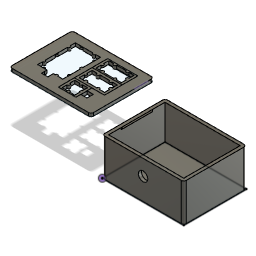
feather_case (Autodesk Fusion 360 design; units mm, degrees)
Autodesk Fusion 360 part; units mm, degrees
sketch "Base" plane through (0, 0, 0) normal (0, 1, 0) x (1, 0, 0) in component "Top"
  line L0 (0, 0) -> (130, 0)
  line L1 (130, 0) -> (130, 100)
  line L2 (130, 100) -> (0, 100)
  line L3 (0, 100) -> (0, 0)
  dimension "d6" = 130
  dimension "d7" = 100
  constraint horizontal L0
  constraint vertical L1
  constraint horizontal L2
  constraint vertical L3
  constraint coincident L0.start L3.end
  measures "d6" distance of L0.start L0.end
  measures "d7" distance of L0.start L2.end
extrude "Extrude1" add sketch "Base" along normal blind 60 makes body 1 in component "Top"
fillet "Fillet1" radius 4 4 edges at (130, 30, 0) (0, 30, 0) (130, 30, -100) (0, 30, -100) on bodies 1 in component "Top"
shell "Shell1" thickness 5 removed faces 1 at (85.3333, 60, -33.3333) on bodies 1 in component "Top"
sketch "Knob" plane through (5, 0, 0) normal (1, 0, 0) x (0, 0, -1) in component "Top"
  line L0 (95, 60) -> (5, 60)
  line L1 (5, 5) -> (95, 5)
  line L2 (25, 60) -> (75, 60)
  line L3 (75, 60) -> (75, 57)
  line L4 (75, 57) -> (25, 57)
  line L5 (25, 57) -> (25, 60)
  line L6 (50, 60) -> (50, 57) construction
  line L7 (5, 60) -> (5, 5)
  line L8 (95, 5) -> (95, 60)
  dimension "d12" = 50
  dimension "d13" = 3
  constraint horizontal L2
  constraint vertical L3
  constraint horizontal L4
  constraint vertical L5
  constraint coincident L0 L2.start
  constraint midpoint L0 L6.start
  constraint midpoint L4 L6.end
  constraint vertical L6
  measures "d12" distance of L3.end L4.end
  measures "d13" distance of L2.end L3.end
extrude "Extrude2" add sketch "Knob" along normal blind 6 draft -45 contours L0 L2 L3 L4 L5 bodies 1 in component "Top"
ref_plane "WorkPlane2" through (65, 30, -50) normal (-1, 0, 0) x (0, 0, 1) in component "Top"
mirror "Mirror1" about plane through (65, 30, -50) normal (-1, 0, 0) of "Extrude2" in component "Top"
sketch "Top" plane through (0, 60, 0) normal (0, 1, 0) x (-1, 0, 0) in component "Base"
  line L0 (-130, -4) -> (-130, -96)
  arc A0 (-130, -96) -> (-126, -100) centre (-126, -96) ccw
  line L1 (-126, -100) -> (-4, -100)
  arc A1 (-4, -100) -> (0, -96) centre (-4, -96) ccw
  line L2 (0, -96) -> (0, -4)
  arc A2 (0, -4) -> (-4, 0) centre (-4, -4) ccw
  line L3 (-4, 0) -> (-126, 0)
  arc A3 (-126, 0) -> (-130, -4) centre (-126, -4) ccw
  line L4 (-125, -25) -> (-125, -5)
  line L5 (-125, -5) -> (-5, -5)
  line L6 (-5, -5) -> (-5, -25)
  line L7 (-5, -25) -> (-5, -75)
  line L8 (-5, -75) -> (-5, -95)
  line L9 (-5, -95) -> (-125, -95)
  line L10 (-125, -75) -> (-125, -25)
  line L11 (-125, -95) -> (-125, -75)
extrude "Extrude1'" add sketch "Top" along normal blind 5 separate body contours L0 A0 L1 A1 L2 A2 L3 A3 | L4 L5 L6 L7 L8 L9 L10 L11 makes body 2 in component "Base"
sketch "Lip" plane through (0, 60, 0) normal (0, -1, 0) x (1, 0, 0) in component "Base"
  arc A0 (130, -4) -> (126, 0) centre (126, -4) ccw
  line L0 (126, 0) -> (4, 0)
  arc A1 (4, 0) -> (0, -4) centre (4, -4) ccw
  line L1 (0, -4) -> (0, -96)
  arc A2 (0, -96) -> (4, -100) centre (4, -96) ccw
  line L2 (4, -100) -> (126, -100)
  arc A3 (126, -100) -> (130, -96) centre (126, -96) ccw
  line L3 (130, -96) -> (130, -4)
  line L4 (124.8, -94.8) -> (124.8, -5.2)
  line L5 (124.8, -5.2) -> (5.2, -5.2)
  line L6 (5.2, -5.2) -> (5.2, -94.8)
  line L7 (5.2, -94.8) -> (124.8, -94.8)
  dimension "d19" = 5.2
extrude "Extrude2'" add sketch "Lip" along normal blind 3 contours L4 L5 L6 L7 bodies 2 in component "Base"
extrude "Extrude3" cut sketch "Knob" along normal blind 3 draft -45 from surface at 0.2 contours L0 L2 L3 L4 L5 bodies 2 in component "Base"
mirror "Mirror1'" about plane through (65, 30, -50) normal (-1, 0, 0) of "Extrude3" in component "Base"
shell "Shell1'" thickness 5 removed faces 1 at (45.0667, 57, -41.6667) on bodies 2 in component "Base"
chamfer "Chamfer1" distance 0.6 angle 45 2 edges at (5.2, 57, -50) (124.8, 57, -50) on bodies 2 in component "Base"
sketch "Sketch3" plane through (0, 0, 0) normal (0, 0, 1) x (1, 0, 0)
  line L0 (4, 60) -> (4, 0)
  line L1 (4, 0) -> (126, 0)
  line L2 (126, 0) -> (126, 60)
  line L3 (126, 60) -> (4, 60)
  circle A0 centre (65, 35) radius 7.5
  line L4 (0, 0) -> (130, 0)
  line L5 (0, 60) -> (0, 0)
  dimension "d55" = 15
  dimension "d56" = 35
  dimension "d57" = 65
  measures "d55" diameter of A0
  measures "d56" distance of A0.centre L4
  measures "d57" distance of A0.centre L5
extrude "Extrude5" cut sketch "Sketch3" against normal blind 5 contours A0 bodies 1 in component "Top"
sketch "Sketch5" plane through (0, 80.6554, 0) normal (0, 1, 0) x (-1, 0, 0)
  arc A0 (21.1976, 0.8625) -> (17.1976, -3.1375) centre (21.1976, -3.1375) ccw
  line L0 (17.1976, -3.1375) -> (17.1976, -95.1375)
  arc A1 (17.1976, -95.1375) -> (21.1976, -99.1375) centre (21.1976, -95.1375) ccw
  line L1 (21.1976, -99.1375) -> (143.1976, -99.1375)
  arc A2 (143.1976, -99.1375) -> (147.1976, -95.1375) centre (143.1976, -95.1375) ccw
  line L2 (147.1976, -95.1375) -> (147.1976, -3.1375)
  arc A3 (147.1976, -3.1375) -> (143.1976, 0.8625) centre (143.1976, -3.1375) ccw
  line L3 (143.1976, 0.8625) -> (21.1976, 0.8625)
  line L4 (131.9976, -88.9375) -> (83.9976, -88.9375)
  line L5 (83.9976, -88.9375) -> (83.9976, -20.9375)
  line L6 (83.9976, -20.9375) -> (131.9976, -20.9375)
  line L7 (131.9976, -20.9375) -> (131.9976, -88.9375)
  line L8 (80.4976, -88.9375) -> (32.4976, -88.9375)
  line L9 (32.4976, -88.9375) -> (32.4976, -35.8375)
  line L10 (32.4976, -35.8375) -> (80.4976, -35.8375)
  line L11 (80.4976, -35.8375) -> (80.4976, -88.9375)
  line L12 (80.4976, -35.8375) -> (52.4976, -35.8375)
  line L13 (52.4976, -35.8375) -> (52.4976, -10.2375)
  line L14 (52.4976, -10.2375) -> (80.4976, -10.2375)
  line L15 (80.4976, -10.2375) -> (80.4976, -35.8375)
  line L16 (112.9976, -20.9375) -> (102.9976, -20.9375)
  line L17 (102.9976, -20.9375) -> (102.9976, -15.9375)
  line L18 (102.9976, -15.9375) -> (112.9976, -15.9375)
  line L19 (112.9976, -15.9375) -> (112.9976, -20.9375)
  line L20 (52.4976, -28.0375) -> (42.4976, -28.0375)
  line L21 (42.4976, -28.0375) -> (42.4976, -18.0375)
  line L22 (42.4976, -18.0375) -> (52.4976, -18.0375)
  line L23 (52.4976, -18.0375) -> (52.4976, -28.0375)
  dimension "d80" = 48
  dimension "d81" = 68
  dimension "d82" = 10.2
  dimension "d83" = 15.2
  dimension "d84" = 48
  dimension "d85" = 53.1
  dimension "d86" = 28
  dimension "d87" = 25.6
  dimension "d88" = 10.2
  dimension "d89" = 15.3
  dimension "d92" = 10
  dimension "d93" = 5
  dimension "d94" = 19
  dimension "d95" = 10
  dimension "d96" = 10
  dimension "d97" = 7.8
  constraint horizontal L4
  constraint vertical L5
  constraint horizontal L6
  constraint vertical L7
  constraint horizontal L8
  constraint vertical L9
  constraint horizontal L10
  constraint vertical L11
  constraint horizontal L12
  constraint vertical L13
  constraint horizontal L14
  constraint vertical L15
  constraint horizontal L16
  constraint vertical L17
  constraint horizontal L18
  constraint vertical L19
  constraint coincident L6 L16.start
  constraint horizontal L20
  constraint vertical L21
  constraint horizontal L22
  constraint vertical L23
  constraint coincident L13 L20.start
  measures "d80" distance of L4.start L4.end
  measures "d81" distance of L4.start L6.end
  measures "d82" distance of L1 L4
  measures "d83" distance of L2 L7
  measures "d84" distance of L8.start L8.end
  measures "d85" distance of L8.start L10.end
  measures "d86" distance of L10.end L12.end
  measures "d87" distance of L10.end L14.end
  measures "d88" distance of L1 L8
  measures "d89" distance of L0 L9
  measures "d92" distance of L16.start L16.end
  measures "d93" distance of L16.start L18.end
  measures "d94" distance of L7 L19
  measures "d95" distance of L20.start L20.end
  measures "d96" distance of L20.start L22.end
  measures "d97" distance of L10 L20
extrude "Extrude6" cut sketch "Sketch5" against normal blind 5 contours L4 L5 L6 L7 L16 | L6 L16 L17 L18 L19 | L8 L9 L10 L11 L12 | L10 L12 L13 L14 L15 L23 | L13 L20 L21 L22 L23 sketch seen with x (1, 0, 0) y (0, 1, 0) z (0, 0, 1) at (147.1976, -15.6554, -0.8625) bodies 2 in component "Base"
sketch "Sketch2" plane through (0, 0, 0) normal (0, 0, 1) x (-1, 0, 0) in component "co2 holder v8"
  line L0 (-34, 24) -> (-34, -24)
  line L1 (-34, -24) -> (34, -24)
  line L2 (34, -24) -> (34, 24)
  line L3 (34, 24) -> (-34, 24)
  line L4 (34.1, 24.1) -> (-34.1, 24.1)
  line L5 (-34.1, 24.1) -> (-34.1, -24.1)
  line L6 (-34.1, -24.1) -> (34.1, -24.1)
  line L7 (34.1, -24.1) -> (34.1, 24.1)
  line L8 (34.1, 24.1) -> (-34.1, -24.1) construction
  line L9 (-34.1, 24.1) -> (34.1, -24.1) construction
  dimension "d5" = 68.2
  dimension "d6_1" = 48.2
  constraint horizontal L4
  constraint perpendicular L4 L5
  constraint parallel L4 L6
  constraint parallel L5 L7
  constraint coincident L8 origin
  constraint coincident L9 origin
  measures "d5" distance of L5.end L6.end
  measures "d6_1" distance of L4.end L5.end
extrude "Extrude2''" add sketch "Sketch2" along normal blind 5 separate body contours L0 L1 L2 L3 | L4 L5 L6 L7 makes body 3 in component "co2 holder v8"
shell "Shell1''" thickness 4 removed faces 2 at (11.3667, 8.0333, 0) at (11.3667, 8.0333, 5) on bodies 3 in component "co2 holder v8"
sketch "pillar sketch" plane through (0, 0, 5) normal (0, 0, 1) x (-1, 0, 0) in component "co2 holder v8"
  line L0 (30.1, -20.1) -> (-30.1, -20.1)
  line L1 (-30.1, -20.1) -> (-30.1, 20.1)
  line L2 (-30.1, 20.1) -> (30.1, 20.1)
  line L3 (30.1, 20.1) -> (30.1, -20.1)
  line L4 (34.1, -24.1) -> (34.1, 24.1)
  line L5 (34.1, 24.1) -> (-34.1, 24.1)
  line L6 (-34.1, 24.1) -> (-34.1, -24.1)
  line L7 (-34.1, -24.1) -> (34.1, -24.1)
  circle A0 centre (0, 19.9) radius 2.1
  circle A1 centre (29.9, 10) radius 2.1
  circle A2 centre (-29.9, 10) radius 2.1
  circle A3 centre (20, -19.9) radius 2.1
  circle A4 centre (-20, -19.9) radius 2.1
  dimension "d11_1" = 4.2
  dimension "d15_1" = 4.2
  dimension "d18_1" = 4.2
  dimension "d23_1" = 0.2
  dimension "d24_1" = 0.2
  dimension "d25_1" = 0.2
  dimension "d27_1" = 4.2
  dimension "d28" = 0.2
  dimension "d29" = 10.1
  dimension "d30" = 10.1
  dimension "d31" = 10.1
  dimension "d32" = 4.2
  dimension "d33" = 0.2
  dimension "d34" = 10.1
  measures "d11_1" diameter of A0
  measures "d15_1" diameter of A1
  measures "d18_1" diameter of A2
  measures "d23_1" distance of L3 A1.centre
  measures "d24_1" distance of L2 A0.centre
  measures "d25_1" distance of L1 A2.centre
  measures "d27_1" diameter of A3
  measures "d28" distance of L0 A3.centre
  measures "d29" distance of L3 A3.centre
  measures "d30" distance of L2 A1.centre
  measures "d31" distance of L2 A2.centre
  measures "d32" diameter of A4
  measures "d33" distance of L0 A4.centre
  measures "d34" distance of L1 A4.centre
extrude "Extrude3'" add sketch "pillar sketch" against normal blind 5 contours L0 A3 | L3 A1 | L0 A4 | L2 A0 | L1 A2 picked at (20.5146, -19.3943) picked at (29.3788, 9.752) picked at (-19.3838, -19.1714) picked at (0.6581, 19.0774) picked at (-29.3932, 10.2832) bodies 3 in component "co2 holder v8"
sketch "hollow sketch A" plane through (0, 0, 5) normal (0, 0, 1) x (-1, 0, 0) in component "co2 holder v8"
  line L0 (30.1, -20.1) -> (22.0905, -20.1)
  arc A0 (22.0905, -20.1) -> (17.9095, -20.1) centre (20, -19.9) ccw
  line L1 (17.9095, -20.1) -> (-17.9095, -20.1)
  arc A1 (-17.9095, -20.1) -> (-22.0905, -20.1) centre (-20, -19.9) ccw
  line L2 (-22.0905, -20.1) -> (-30.1, -20.1)
  line L3 (-30.1, -20.1) -> (-30.1, 7.9095)
  arc A2 (-30.1, 7.9095) -> (-30.1, 12.0905) centre (-29.9, 10) ccw
  line L4 (-30.1, 12.0905) -> (-30.1, 20.1)
  line L5 (-30.1, 20.1) -> (-2.0905, 20.1)
  arc A3 (-2.0905, 20.1) -> (2.0905, 20.1) centre (0, 19.9) ccw
  line L6 (2.0905, 20.1) -> (30.1, 20.1)
  line L7 (30.1, 20.1) -> (30.1, 12.0905)
  arc A4 (30.1, 12.0905) -> (30.1, 7.9095) centre (29.9, 10) ccw
  line L8 (30.1, 7.9095) -> (30.1, -20.1)
  line L9 (34.1, -24.1) -> (34.1, 24.1)
  line L10 (34.1, 24.1) -> (-34.1, 24.1)
  line L11 (-34.1, 24.1) -> (-34.1, -24.1)
  line L12 (-34.1, -24.1) -> (34.1, -24.1)
  circle A5 centre (20, 20.3) radius 2.1
  circle A6 centre (30.3, -10) radius 2.1
  circle A7 centre (-30.3, -10) radius 2.1
  circle A8 centre (0, -20.3) radius 2.1
  circle A9 centre (-20, 20.3) radius 2.1
  dimension "d37" = 4.2
  dimension "d38" = 4.2
  dimension "d39" = 4.2
  dimension "d40" = 4.2
  dimension "d41" = 4.2
  dimension "d42" = 0.2
  dimension "d44" = 0.2
  dimension "d45" = 10.1
  dimension "d46" = 10.1
  dimension "d47" = 10.1
  dimension "d49" = 10.1
  dimension "d51" = 0.2
  measures "d37" diameter of A5
  measures "d38" diameter of A6
  measures "d39" diameter of A7
  measures "d40" diameter of A8
  measures "d41" diameter of A9
  measures "d42" distance of L1 A8.centre
  measures "d44" distance of L3 A7.centre
  measures "d45" distance of L2 A7.centre
  measures "d46" distance of L0 A6.centre
  measures "d47" distance of L7 A5.centre
  measures "d49" distance of L4 A9.centre
  measures "d51" distance of L5 A9.centre
extrude "Extrude4" add sketch "hollow sketch A" against normal blind 3 from surface at -2 contours L8 A6 | L1 A8 | L6 A5 | L3 A7 | L5 A9 picked at (29.4743, -9.8971) picked at (-0.2209, -19.3952) picked at (20.5114, 18.7272) picked at (-28.7439, -10.2036) picked at (-20.6202, 19.3298) bodies 3 in component "co2 holder v8"
extrude "Extrude5'" cut sketch "hollow sketch A" against normal blind 2 contours L8 A6 | L1 A8 | L1 A8 | L6 A5 | L6 A5 | L3 A7 | L3 A7 | L5 A9 | L5 A9 picked at (30.8398, -9.8081) bodies 3 in component "co2 holder v8"
sketch "Sketch1" plane through (0, 0, 0) normal (0, 0, 1) x (1, 0, 0) in component "2x1 case v3 (1)"
  line L0 (24.2, -14.2) -> (-24.2, -14.2)
  line L1 (-24.2, -14.2) -> (-24.2, 14.2)
  line L2 (-24.2, 14.2) -> (24.2, 14.2)
  line L3 (24.2, 14.2) -> (24.2, -14.2)
  line L4 (24.2, -14.2) -> (-24.2, 14.2) construction
  line L5 (-24.2, -14.2) -> (24.2, 14.2) construction
  dimension "d1_2" = 48.4
  dimension "d2_2" = 28.4
  constraint horizontal L0
  constraint perpendicular L0 L1
  constraint parallel L0 L2
  constraint parallel L1 L3
  constraint coincident L4 origin
  constraint coincident L5 origin
  measures "d1_2" distance of L1.end L2.end
  measures "d2_2" distance of L0 L2
extrude "Extrude1''" add sketch "Sketch1" along normal blind 5 separate body makes body 4 in component "2x1 case v3 (1)"
shell "Shell1'''" thickness 4 removed faces 2 at (-8.0667, 4.7333, 5) at (-8.0667, 4.7333, 0) on bodies 4 in component "2x1 case v3 (1)"
sketch "Sketch2 (2)" plane through (0, 0, 5) normal (0, 0, 1) x (-1, 0, 0) in component "2x1 case v3 (1)"
  line L0 (-20.2, -10.2) -> (-20.2, 10.2)
  line L1 (-20.2, 10.2) -> (20.2, 10.2)
  line L2 (20.2, 10.2) -> (20.2, -10.2)
  line L3 (20.2, -10.2) -> (-20.2, -10.2)
  line L4 (-24.2, -14.2) -> (24.2, -14.2)
  line L5 (24.2, -14.2) -> (24.2, 14.2)
  line L6 (24.2, 14.2) -> (-24.2, 14.2)
  line L7 (-24.2, 14.2) -> (-24.2, -14.2)
  circle A0 centre (19.9, 0) radius 2.1
  circle A1 centre (10, -9.9) radius 2.4
  circle A2 centre (-10, -9.9) radius 2.1
  circle A3 centre (-19.9, 0) radius 2.4
  line L8 (-20.2, 0) -> (20.2, 0) construction
  line L9 (0, -10.2) -> (0, 10.2) construction
  circle A4 centre (-10, 9.9) radius 2.1
  circle A5 centre (10, 9.9) radius 2.4
  dimension "d6_3" = 4.2
  dimension "d7_3" = 0.3
  dimension "d8_3" = 4.8
  dimension "d9_3" = 0.3
  dimension "d11_3" = 4.2
  dimension "d12_2" = 0.3
  dimension "d14_2" = 4.8
  dimension "d15_3" = 0.3
  dimension "d16_2" = 10
  dimension "d17_2" = 10
  dimension "d18_3" = 4.2
  dimension "d19_2" = 0.3
  dimension "d20_2" = 10
  dimension "d21_2" = 4.8
  dimension "d22_2" = 10
  dimension "d23_3" = 0.3
  constraint midpoint L0 L8.start
  constraint midpoint L2 L8.end
  constraint midpoint L3 L9.start
  constraint midpoint L1 L9.end
  measures "d6_3" diameter of A0
  measures "d7_3" distance of L2 A0.centre
  measures "d8_3" diameter of A1
  measures "d9_3" distance of L3 A1.centre
  measures "d11_3" diameter of A2
  measures "d12_2" distance of L3 A2.centre
  measures "d14_2" diameter of A3
  measures "d15_3" distance of L0 A3.centre
  measures "d16_2" distance of A2.centre L9
  measures "d17_2" distance of A1.centre L9
  measures "d18_3" diameter of A4
  measures "d19_2" distance of L1 A4.centre
  measures "d20_2" distance of L9 A4.centre
  measures "d21_2" diameter of A5
  measures "d22_2" distance of L9 A5.centre
  measures "d23_3" distance of L1 A5.centre
extrude "Extrude2'''" add sketch "Sketch2 (2)" against normal blind 5 contours L0 A3 | L3 A1 | L1 A5 picked at (-19.3318, 0.2231) picked at (10.663, -9.6523) picked at (9.8572, 8.5699) bodies 4 in component "2x1 case v3 (1)"
extrude "Extrude3''" cut sketch "Sketch2 (2)" against normal blind 2 contours L3 A2 | L1 A4 | L2 A0 picked at (-9.7306, -10.8343) picked at (-9.8029, 10.7717) picked at (20.689, 0.3783) bodies 4 in component "2x1 case v3 (1)"
extrude "Extrude4'" add sketch "Sketch2 (2)" against normal blind 3 from surface at -2 contours L3 A2 | L1 A4 | L2 A0 picked at (-9.4862, -9.6246) picked at (-9.5626, 9.5535) picked at (19.4174, 0.1552) bodies 4 in component "2x1 case v3 (1)"
sketch "Sketch1 (2)" plane through (0, 0, 0) normal (0, 0, 1) x (1, 0, 0) in component "2x1 case v3"
  line L0 (24.2, -14.2) -> (-24.2, -14.2)
  line L1 (-24.2, -14.2) -> (-24.2, 14.2)
  line L2 (-24.2, 14.2) -> (24.2, 14.2)
  line L3 (24.2, 14.2) -> (24.2, -14.2)
  line L4 (24.2, -14.2) -> (-24.2, 14.2) construction
  line L5 (-24.2, -14.2) -> (24.2, 14.2) construction
  dimension "d1_1" = 48.4
  dimension "d2_1" = 28.4
  constraint horizontal L0
  constraint perpendicular L0 L1
  constraint parallel L0 L2
  constraint parallel L1 L3
  constraint coincident L4 origin
  constraint coincident L5 origin
  measures "d1_1" distance of L1.end L2.end
  measures "d2_1" distance of L0 L2
extrude "Extrude1'''" add sketch "Sketch1 (2)" along normal blind 5 separate body makes body 5 in component "2x1 case v3"
shell "Shell1''''" thickness 4 removed faces 2 at (-8.0667, 4.7333, 5) at (-8.0667, 4.7333, 0) on bodies 5 in component "2x1 case v3"
sketch "Sketch2 (3)" plane through (0, 0, 5) normal (0, 0, 1) x (-1, 0, 0) in component "2x1 case v3"
  line L0 (-20.2, -10.2) -> (-20.2, 10.2)
  line L1 (-20.2, 10.2) -> (20.2, 10.2)
  line L2 (20.2, 10.2) -> (20.2, -10.2)
  line L3 (20.2, -10.2) -> (-20.2, -10.2)
  line L4 (-24.2, -14.2) -> (24.2, -14.2)
  line L5 (24.2, -14.2) -> (24.2, 14.2)
  line L6 (24.2, 14.2) -> (-24.2, 14.2)
  line L7 (-24.2, 14.2) -> (-24.2, -14.2)
  circle A0 centre (19.9, 0) radius 2.1
  circle A1 centre (10, -9.9) radius 2.4
  circle A2 centre (-10, -9.9) radius 2.1
  circle A3 centre (-19.9, 0) radius 2.4
  line L8 (-20.2, 0) -> (20.2, 0) construction
  line L9 (0, -10.2) -> (0, 10.2) construction
  circle A4 centre (-10, 9.9) radius 2.1
  circle A5 centre (10, 9.9) radius 2.4
  dimension "d6_2" = 4.2
  dimension "d7_2" = 0.3
  dimension "d8_2" = 4.8
  dimension "d9_2" = 0.3
  dimension "d11_2" = 4.2
  dimension "d12_1" = 0.3
  dimension "d14_1" = 4.8
  dimension "d15_2" = 0.3
  dimension "d16_1" = 10
  dimension "d17_1" = 10
  dimension "d18_2" = 4.2
  dimension "d19_1" = 0.3
  dimension "d20_1" = 10
  dimension "d21_1" = 4.8
  dimension "d22_1" = 10
  dimension "d23_2" = 0.3
  constraint midpoint L0 L8.start
  constraint midpoint L2 L8.end
  constraint midpoint L3 L9.start
  constraint midpoint L1 L9.end
  measures "d6_2" diameter of A0
  measures "d7_2" distance of L2 A0.centre
  measures "d8_2" diameter of A1
  measures "d9_2" distance of L3 A1.centre
  measures "d11_2" diameter of A2
  measures "d12_1" distance of L3 A2.centre
  measures "d14_1" diameter of A3
  measures "d15_2" distance of L0 A3.centre
  measures "d16_1" distance of A2.centre L9
  measures "d17_1" distance of A1.centre L9
  measures "d18_2" diameter of A4
  measures "d19_1" distance of L1 A4.centre
  measures "d20_1" distance of L9 A4.centre
  measures "d21_1" diameter of A5
  measures "d22_1" distance of L9 A5.centre
  measures "d23_2" distance of L1 A5.centre
extrude "Extrude2''''" add sketch "Sketch2 (3)" against normal blind 5 contours L0 A3 | L3 A1 | L1 A5 picked at (-19.3318, 0.2231) picked at (10.663, -9.6523) picked at (9.8572, 8.5699) bodies 5 in component "2x1 case v3"
extrude "Extrude3'''" cut sketch "Sketch2 (3)" against normal blind 2 contours L3 A2 | L1 A4 | L2 A0 picked at (-9.7306, -10.8343) picked at (-9.8029, 10.7717) picked at (20.689, 0.3783) bodies 5 in component "2x1 case v3"
extrude "Extrude4''" add sketch "Sketch2 (3)" against normal blind 3 from surface at -2 contours L3 A2 | L1 A4 | L2 A0 picked at (-9.4862, -9.6246) picked at (-9.5626, 9.5535) picked at (19.4174, 0.1552) bodies 5 in component "2x1 case v3"
sketch "Sketch1 (3)" plane through (0, 0, 0) normal (0, 0, 1) x (1, 0, 0) in component "1x1 case v2"
  line L0 (14.2, -14.2) -> (-14.2, -14.2)
  line L1 (-14.2, -14.2) -> (-14.2, 14.2)
  line L2 (-14.2, 14.2) -> (14.2, 14.2)
  line L3 (14.2, 14.2) -> (14.2, -14.2)
  line L4 (14.2, -14.2) -> (-14.2, 14.2) construction
  line L5 (-14.2, -14.2) -> (14.2, 14.2) construction
  dimension "d1_3" = 28.4
  dimension "d2_3" = 28.4
  constraint horizontal L0
  constraint perpendicular L0 L1
  constraint parallel L0 L2
  constraint parallel L1 L3
  constraint coincident L4 origin
  constraint coincident L5 origin
  measures "d1_3" distance of L1.end L2.end
  measures "d2_3" distance of L0 L2
extrude "Extrude1''''" add sketch "Sketch1 (3)" along normal blind 5 separate body makes body 6 in component "1x1 case v2"
shell "Shell1'''''" thickness 4 removed faces 2 at (-4.7333, 4.7333, 5) at (-4.7333, 4.7333, 0) on bodies 6 in component "1x1 case v2"
sketch "Sketch2 (4)" plane through (0, 0, 5) normal (0, 0, 1) x (-1, 0, 0) in component "1x1 case v2"
  line L0 (-10.2, -10.2) -> (-10.2, 10.2)
  line L1 (-10.2, 10.2) -> (10.2, 10.2)
  line L2 (10.2, 10.2) -> (10.2, -10.2)
  line L3 (10.2, -10.2) -> (-10.2, -10.2)
  line L4 (-14.2, -14.2) -> (14.2, -14.2)
  line L5 (14.2, -14.2) -> (14.2, 14.2)
  line L6 (14.2, 14.2) -> (-14.2, 14.2)
  line L7 (-14.2, 14.2) -> (-14.2, -14.2)
  circle A0 centre (0, -9.9) radius 2.1
  circle A1 centre (-9.9, 0) radius 2.4
  line L8 (-10.2, 0) -> (10.2, 0) construction
  line L9 (0, -10.2) -> (0, 10.2) construction
  circle A2 centre (0, 9.9) radius 2.1
  circle A3 centre (9.9, 0) radius 2.4
  line L10 (-9, 2.2249) -> (-9, -2.2249)
  dimension "d11_4" = 4.2
  dimension "d12_3" = 0.3
  dimension "d14_3" = 4.8
  dimension "d15_4" = 0.3
  dimension "d18_4" = 4.2
  dimension "d19_3" = 0.3
  dimension "d21_3" = 4.8
  dimension "d31_1" = 0.3
  dimension "d110" = 0.9
  constraint midpoint L0 L8.start
  constraint midpoint L2 L8.end
  constraint midpoint L3 L9.start
  constraint midpoint L1 L9.end
  constraint coincident A0.centre L9
  constraint coincident L9 A2.centre
  constraint coincident L8 A3.centre
  constraint coincident A1 L10.start
  constraint coincident A1 L10.end
  constraint parallel L0 L10
  measures "d11_4" diameter of A0
  measures "d12_3" distance of L3 A0.centre
  measures "d14_3" diameter of A1
  measures "d15_4" distance of L0 A1.centre
  measures "d18_4" diameter of A2
  measures "d19_3" distance of L1 A2.centre
  measures "d21_3" diameter of A3
  measures "d31_1" distance of L2 A3.centre
  measures "d110" distance of A1.centre L10
extrude "Extrude2'''''" add sketch "Sketch2 (4)" against normal blind 5 contours L0 A1 L10 | L2 A3 picked at (9.3022, -0.0589) bodies 6 in component "1x1 case v2"
extrude "Extrude3''''" cut sketch "Sketch2 (4)" against normal blind 2 contours L3 A0 | L1 A2 picked at (0.2907, -10.7368) picked at (-0.1971, 10.7717) bodies 6 in component "1x1 case v2"
extrude "Extrude4'''" add sketch "Sketch2 (4)" against normal blind 3 from surface at -2 contours L3 A0 | L1 A2 picked at (0.2572, -9.449) picked at (0.2572, 9.449) bodies 6 in component "1x1 case v2"
move_body "Move1" bodies 3 to x (1, 0, 0) y (0, 1, 0) z (0, 0, 1) at (0, 0, 2.8117) in component "co2 holder v8"
move_body "Move1'" bodies 5 to x (1, 0, 0) y (0, 1, 0) z (0, 0, 1) at (0, 0, 0.0188) in component "2x1 case v3"
move_body "Move1''" bodies 4 to x (1, 0, 0) y (0, 1, 0) z (0, 0, 1) at (0, 0, 0.0188) in component "2x1 case v3 (1)"
move_body "Move1'''" bodies 6 to x (1, 0, 0) y (0, 1, 0) z (0, 0, 1) at (0, 0, 0.0188) in component "1x1 case v2"
move_body "Move2" bodies 6 to x (1, 0, 0) y (0, 1, 0) z (0, 0, 1) at (0, 0, 0.0007) in component "1x1 case v2"
move_body "Move2'" bodies 5 to x (1, 0, 0) y (0, 1, 0) z (0, 0, 1) at (0, 0, -0.0009) in component "2x1 case v3"
sketch "Sketch7" plane through (0, 80.6554, 0) normal (0, 1, 0) x (-1, 0, 0)
  line L0 (128.1105, -24.8223) -> (128.1105, -32.8319)
  arc A0 (128.1105, -32.8319) -> (128.1105, -37.0128) centre (127.9105, -34.9223) ccw
  line L1 (128.1105, -37.0128) -> (128.1105, -52.8319)
  line L2 (128.1105, -52.8319) -> (128.1105, -57.0128)
  line L3 (128.1105, -57.0128) -> (128.1105, -72.8319)
  arc A1 (128.1105, -72.8319) -> (128.1105, -77.0128) centre (127.9105, -74.9223) ccw
  line L4 (128.1105, -77.0128) -> (128.1105, -85.0223)
  line L5 (128.1105, -85.0223) -> (120.101, -85.0223)
  line L6 (120.101, -85.0223) -> (115.9201, -85.0223)
  line L7 (115.9201, -85.0223) -> (100.101, -85.0223)
  arc A2 (100.101, -85.0223) -> (95.9201, -85.0223) centre (98.0105, -84.8223) ccw
  line L8 (95.9201, -85.0223) -> (87.9105, -85.0223)
  line L9 (87.9105, -85.0223) -> (87.9105, -77.0128)
  line L10 (87.9105, -77.0128) -> (87.9105, -72.8319)
  line L11 (87.9105, -72.8319) -> (87.9105, -57.0128)
  arc A3 (87.9105, -57.0128) -> (87.9105, -52.8319) centre (88.1105, -54.9223) ccw
  line L12 (87.9105, -52.8319) -> (87.9105, -37.0128)
  line L13 (87.9105, -37.0128) -> (87.9105, -32.8319)
  line L14 (87.9105, -32.8319) -> (87.9105, -24.8223)
  line L15 (87.9105, -24.8223) -> (95.9201, -24.8223)
  arc A4 (95.9201, -24.8223) -> (100.101, -24.8223) centre (98.0105, -25.0223) ccw
  line L16 (100.101, -24.8223) -> (115.9201, -24.8223)
  line L17 (115.9201, -24.8223) -> (120.101, -24.8223)
  line L18 (120.101, -24.8223) -> (128.1105, -24.8223)
  line L19 (83.9105, -89.0223) -> (132.1105, -89.0223)
  line L20 (132.1105, -89.0223) -> (132.1105, -20.8223)
  line L21 (132.1105, -20.8223) -> (83.9105, -20.8223)
  line L22 (83.9105, -20.8223) -> (83.9105, -89.0223)
  line L23 (103.0975, -20.8223) -> (113.0975, -20.8223)
  line L24 (113.0975, -20.8223) -> (113.0975, -24.8223)
  line L25 (113.0975, -24.8223) -> (103.0975, -24.8223)
  line L26 (103.0975, -24.8223) -> (103.0975, -20.8223)
  dimension "d103" = 10
  dimension "d104" = 4
  dimension "d105" = 19.187
  constraint horizontal L23
  constraint vertical L24
  constraint horizontal L25
  constraint vertical L26
  constraint coincident L21 L23.start
  measures "d103" distance of L23.start L23.end
  measures "d104" distance of L23.start L25.end
  measures "d105" distance of L22 L26
extrude "Extrude8" cut sketch "Sketch7" against normal blind 5 contours L16 L21 L23 L24 L25 L26 sketch seen with x (1, 0, 0) y (0, 1, 0) z (0, 0, 1) at (147.1976, -15.6554, -0.8625) bodies 2 in component "Base"
extrude "Extrude8'" cut sketch "Sketch7" against normal blind 5 contours L16 L21 L23 L24 L25 L26 sketch seen with x (0, -1, 0) y (0, 0, -1) z (1, 0, 0) at (54.9223, -108.0105, 83.4671) bodies 3 in component "co2 holder v8"
combine "Combine2" operation add target body 2 tool bodies 3 4 5 6 body 3 seen with x (0, 0, 1) y (-1, 0, 0) z (0, -1, 0) at (39.187, 67.8117, -55.7848) body 4 seen with x (1, 0, 0) y (0, 0, 1) z (0, -1, 0) at (90.6976, 65.0179, -77.5892) body 5 seen with x (1, 0, 0) y (0, 0, 1) z (0, -1, 0) at (90.6976, 65.0179, -50.8892) body 6 seen with x (1, 0, 0) y (0, 0, 1) z (0, -1, 0) at (80.6976, 65.0194, -23.3876) in component "Base"
component "Enclosure" placed x (1, 0, 0) y (0, 1, 0) z (0, 0, 1) at (0, 0, 0)
component "co2 holder v8" placed x (0, 0, 1) y (-1, 0, 0) z (0, -1, 0) at (-108.0105, 83.4671, -54.9223)
component "2x1 case v3 (1)" placed x (1, 0, 0) y (0, 0, 1) z (0, -1, 0) at (-56.5, 80.6733, -76.7267)
component "2x1 case v3" placed x (1, 0, 0) y (0, 0, 1) z (0, -1, 0) at (-56.5, 80.6733, -50.0267)
component "1x1 case v2" placed x (1, 0, 0) y (0, 0, 1) z (0, -1, 0) at (-66.5, 80.6749, -22.5251)
component "Top" placed x (1, 0, 0) y (0, 1, 0) z (0, 0, 1) at (0, 0, 0) in component "Enclosure"
component "Base" placed x (1, 0, 0) y (0, 1, 0) z (0, 0, 1) at (-147.1976, 15.6554, 0.8625) in component "Enclosure"
equation "Width = 100 mm"
equation "length = 130 mm"
equation "heigth = 60 mm"
equation "shell = 5 mm"
equation "gap = 0.2 mm"
equation "d6 = length"
equation "d7 = Width"
equation "d8 = heigth"
equation "d11 = shell"
equation "d12 = Width / 2"
equation "d17 = shell"
equation "d19 = shell + gap"
equation "d26 = shell"
equation "d57 = length / 2"
equation "d5 = 68 mm + space_error * 2"
equation "d6_1 = 48 mm + space_error * 2"
equation "error_hollow = 0.2 mm" comment "das wo e ussparig isch, grechnet vom innere rand"
equation "d11_1 = diam_pillar"
equation "diam_hollow = 4.2 mm" comment "das wo e ussparig isch, dr durchmesser"
equation "error_pillar = 0.2 mm" comment "das wo ine e sühle isch, grechnet vom innere rand"
equation "diam_pillar = 4.2 mm" comment "das wo ine e sühle isch, dr durchmesser"
equation "d15_1 = diam_pillar"
equation "d18_1 = diam_pillar"
equation "d23_1 = error_pillar"
equation "d24_1 = error_pillar"
equation "d25_1 = error_pillar"
equation "d27_1 = diam_pillar"
equation "d28 = error_pillar"
equation "d29 = 10 mm + space_error"
equation "d30 = 10 mm + space_error"
equation "d31 = 10 mm + space_error"
equation "d32 = diam_pillar"
equation "d33 = error_pillar"
equation "d34 = 10 mm + space_error"
equation "d37 = diam_hollow"
equation "d38 = diam_hollow"
equation "d39 = diam_hollow"
equation "d40 = diam_hollow"
equation "d41 = diam_hollow"
equation "d42 = error_hollow"
equation "d44 = error_hollow"
equation "d45 = 10 mm + space_error"
equation "d46 = 10 mm + space_error"
equation "d47 = 10 mm + space_error"
equation "space_error = 0.1 mm"
equation "d49 = 10 mm + space_error"
equation "d50 = -error_hollow"
equation "d51 = error_hollow"
equation "d66 = -error_hollow"
